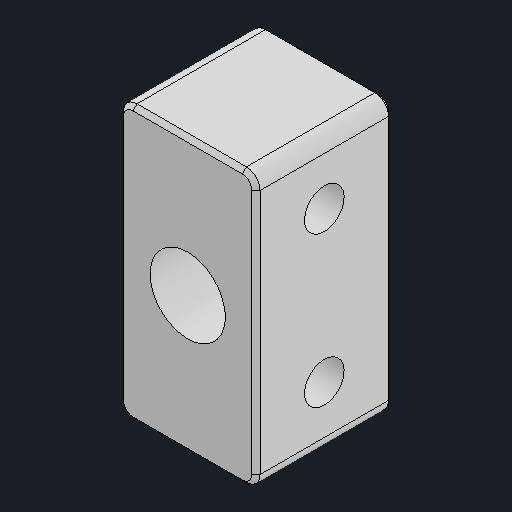
# Autodesk Inventor part: 2020-perp-connecdtor
Saved by Autodesk Inventor 2026 (Build 300175050, 175E)
## iProperties
Created: 2026-01-22
Part Number: 2020-perp-connecdtor
Material: Generic
Document SubType Name: Modeling
Designer: queezz
Density: 1 g/cm^3
Appearance: Default
Author: queezz
Autodesk Inventor part; units mm, degrees
ref_plane "YZ Plane" through (0, 0, 0) normal (1, 0, 0) x (0, 1, 0)
ref_plane "XZ Plane" through (0, 0, 0) normal (0, 1, 0) x (-1, 0, 0)
ref_plane "XY Plane" through (0, 0, 0) normal (0, 0, 1) x (1, 0, 0)
sketch "Sketch7" plane through (0, 0, 0) normal (0, 0, 1) x (1, 0, 0)
  line L0 (0, 0) -> (0, 20)
  line L1 (-20, 0) -> (0, 0)
  line L2 (-20, 8) -> (-8, 8)
  line L3 (-8, 8) -> (-8, 20)
  line L4 (-8, 8) -> (0, 0)
  line L5 (0, 20) -> (-8, 20)
  line L6 (-20, 0) -> (-20, 8)
  dimension "d40" = 20
  dimension "d43" = 45
  dimension "d44" = 8
  constraints: 14 end point, 3 perpendicular, 2 horizontal, 2 vertical, 1 coincident
  measures "d40" distance of L0.start L0.end
  measures "d43" angle of L1 L4
  measures "d44" distance between parallel lines of L1 L2
extrude "Extrusion4" add sketch "Sketch7" along normal mid plane 40
sketch "Sketch8" plane through (-8, 8, 20) normal (-1, 0, 0) x (0, 0, 1)
  line L0 (-31, 2) -> (-9, 2) construction
  line L1 (-40, -8) -> (0, -8) projected
  point P0 (-20, -8)
  point P1 (-20, 2)
  point P2 (-20, -8)
  dimension "d45" = 10
  dimension "d53" = 22
  constraints: 2 coincident, 2 end point, 2 midpoint, 1 horizontal, 1 vertical alignment
  measures "d45" distance between parallel lines of L1 L0
  measures "d53" distance of L0.start L0.end
hole "Hole3" at (-8, 10, -11) at (-8, 10, 11) direction (1, 0, 0) diameter 5.8 end through all
sketch "Sketch9" plane through (-20, 0, 20) normal (0, -1, 0) x (1, 0, 0)
  line L0 (20, 0) -> (20, -40) projected
  point P0 (20, -20)
  point P1 (10, -20)
  point P2 (20, -20)
  point P3 (20, -20)
  dimension "d54" = 10
  constraints: 2 midpoint, 1 horizontal alignment
  measures "d54" distance of point (20, -20) point (10, -20)
hole "Hole4" at (-10, 0, 0) direction (0, 1, 0) diameter 5.8 end through all
sketch "Sketch10" plane through (0, 0, 0) normal (0, 0, 1) x (1, 0, 0)
  line L0 (0, 20) -> (0, 0) projected
  line L1 (0, 0) -> (-20, 0) projected
  line L2 (-20, 0) -> (-20, 20)
  line L3 (-20, 20) -> (0, 20)
  line L4 (0, 20) -> (0, 0) projected
  line L5 (0, 0) -> (-20, 0) projected
  line L6 (-20, 0) -> (-20, 8) projected
  line L7 (-20, 8) -> (-8, 8) projected
  line L8 (-8, 8) -> (-8, 20) projected
  line L9 (-8, 20) -> (0, 20) projected
  constraints: 4 end point, 1 horizontal, 1 vertical
extrude "Extrusion5" add sketch "Sketch10" along normal mid plane 40 contours L8 L7 L2 L3
sketch "Sketch11" plane through (-10, 8, 0) normal (0, -1, 0) x (0, 0, 1)
  circle A0 centre (0, 0) radius 2.9 projected
  point P0 (0, -10)
  point P1 (0, 0)
  constraints: 1 coincident
hole "Hole5" at (-10, 8, 0) direction (0, 1, 0) diameter 11 end through all
sketch "Sketch12" plane through (-8, 10, 11) normal (1, 0, 0) x (0, 0, -1)
  circle A0 centre (22, 0) radius 2.9 projected
  circle A1 centre (0, 0) radius 2.9 projected
  point P0 (11, -10)
  constraints: 2 coincident
hole "Hole6" at (-8, 10, -11) at (-8, 10, 11) direction (-1, 0, 0) diameter 11 end through all
fillet "Fillet4" radius 2 4 edges at (0, 10, 20) (-20, 10, 20) (0, 10, -20) (-20, 10, -20)
chamfer "Chamfer3" distance 0.6 angle 45 14 edges at (-20, 20, 0) (-10, 20, 20) (-0.5858, 20, 19.4142) (0, 20, 0) (-0.5858, 20, -19.4142) (-10, 20, -20) (-20, 0, 0) (-19.4142, 0, 19.4142) (-10, 0, 20) (-0.5858, 0, 19.4142) (0, 0, 0) (-0.5858, 0, -19.4142) (-10, 0, -20) (-19.4142, 0, -19.4142)
chamfer "Chamfer4" distance 0.6 angle 45 1 edges at (-10, 0, 2.9)
move or copy body "Move Body1" bodies to move or copy 1 copy no rotation origin (0, 0, 0) rotation axis (1, 0, 0) rotation angle 90
body "Solid2"
